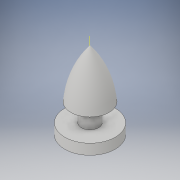
# Autodesk Inventor part: MotorMountingHub
Saved by Autodesk Inventor 2018 (Build 220112000, 112)
## iProperties
Created: 2019-06-13
Part Number: MotorMountingHub
Material: Generic
Document SubType Name: Modeling
Designer: anirudh
Density: 1 g/cm^3
Appearance: Default
Author: anirudh
Autodesk Inventor part; units mm, degrees
ref_plane "YZ Plane" through (0, 0, 0) normal (1, 0, 0) x (0, 1, 0)
ref_plane "XZ Plane" through (0, 0, 0) normal (0, 1, 0) x (-1, 0, 0)
ref_plane "XY Plane" through (0, 0, 0) normal (0, 0, 1) x (1, 0, 0)
sketch "Sketch1" plane through (0, 0, 0) normal (0, 1, 0) x (-1, 0, 0)
  circle A0 centre (0, 0) radius 7.25
  dimension "d0" = 14.5
  constraints: 1 centre point, 1 coincident
  measures "d0" diameter of A0
extrude "Extrusion1" add sketch "Sketch1" along normal blind 3
sketch "Sketch2" plane through (0, 3, 0) normal (0, 1, 0) x (1, 0, 0)
  circle A0 centre (0, 0) radius 2.5
  dimension "d3" = 5
  constraints: 1 centre point, 1 coincident
  measures "d3" diameter of A0
extrude "Extrusion2" add sketch "Sketch2" along normal blind 14.7
ref_plane "Work Plane1" through (0, 8.3, 0) normal (0, 1, 0) x (1, 0, 0)
sketch "Sketch4" plane through (0, 0, 0) normal (0, 0, 1) x (1, 0, 0)
  line L0 (0, 0) -> (0, 8.2998)
  line L1 (0, 8.2998) -> (-5.5, 8.2998)
  line L2 (2.5, 17.7) -> (-2.5, 17.7) projected
  line L3 (0, 22.2998) -> (0, 8.2998)
  arc A0 (0, 22.2998) -> (-5.5, 8.2998) centre (20.0135, 6.357) ccw
  line L4 (0, 22.2998) -> (0, 30.2311)
  dimension "d8" = 5.5
  dimension "d9" = 14
  constraints: 8 end point, 2 perpendicular, 2 point on circle, 2 vertical, 1 centre point
  measures "d8" distance of L0.end L1.end
  measures "d9" distance of L0.end L3.start
revolve "Revolution1" add sketch "Sketch4" angle 360 about axis through (0, 22.2998, 0) along (0, 1, 0)
body "Solid1"
